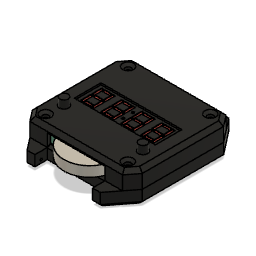
Digital_Watch_Case (Autodesk Fusion 360 design; units mm, degrees)
Autodesk Fusion 360 part; units mm, degrees
sketch "Sketch1" plane through (0, 0, 0) normal (0, 1, 0) x (1, 0, 0)
  line L0 (0, 0) -> (0, 18.5)
  line L1 (0, 18.5) -> (19.75, 18.5)
  line L2 (19.75, 18.5) -> (-19.75, 18.5)
  line L3 (-19.75, 18.5) -> (-19.75, -18.5)
  line L4 (-19.75, -18.5) -> (19.75, -18.5)
  line L5 (19.75, -18.5) -> (19.75, 18.5)
  line L6 (0, 18.5) -> (0, 5.15)
  line L7 (19.75, 0) -> (15.95, 0)
  line L8 (-19.75, 0) -> (-15.95, 0)
  line L9 (0, 5.15) -> (0, -5.05)
  line L10 (-15.95, 0) -> (-15.95, 5.15)
  line L11 (-15.95, 5.15) -> (15.95, 5.15)
  line L12 (15.95, 5.15) -> (15.95, -5.05)
  line L13 (15.95, -5.05) -> (-15.95, -5.05)
  line L14 (-15.95, -5.05) -> (-15.95, 5.15)
  circle A0 centre (0, -15.3) radius 10.25
  line L15 (15.95, -5.05) -> (15.95, -9.75)
  line L16 (19.75, -9.75) -> (15.75, -9.75)
  circle A1 centre (15.75, -9.75) radius 1.665
  circle A2 centre (-15.75, -9.75) radius 1.665
  line L17 (19.75, 18.5) -> (19.75, 17.8)
  line L18 (19.75, 17.8) -> (17.75, 17.8)
  line L19 (17.75, 17.8) -> (15.05, 17.8)
  line L20 (15.05, 17.8) -> (15.05, 15.1)
  line L21 (15.05, 15.1) -> (17.75, 15.1)
  line L22 (17.75, 15.1) -> (17.75, 17.8)
  circle A3 centre (16.4, 16.45) radius 1.35
  circle A4 centre (-16.4, 16.45) radius 1.35
  circle A5 centre (16.4, -16.45) radius 1.35
  circle A6 centre (-16.4, -16.45) radius 1.35
  line L23 (19.75, 18.5) -> (19.75, 15.5)
  line L24 (19.75, 18.5) -> (17.42, 18.5)
  line L25 (17.42, 18.5) -> (19.75, 15.5)
  line L26 (-17.42, 18.5) -> (-19.75, 15.5)
  line L27 (-17.42, -18.5) -> (-19.75, -15.5)
  line L28 (17.42, -18.5) -> (19.75, -15.5)
  line L29 (19.75, 5.15) -> (-19.75, 5.15)
  line L30 (-19.75, 5.15) -> (-19.75, 13.65)
  line L31 (-19.75, 13.65) -> (19.75, 13.65)
  line L32 (19.75, 13.65) -> (19.75, 5.15)
  line L33 (-19.75, 13.65) -> (-9.75, 13.65)
  line L34 (-9.75, 13.65) -> (-19.75, 13.65)
  line L35 (-19.75, 13.65) -> (-19.75, 5.15)
  line L36 (-19.75, 5.15) -> (-9.75, 5.15)
  line L37 (-9.75, 5.15) -> (-9.75, 13.65)
  line L38 (19.75, 13.65) -> (-6.25, 13.65)
  line L39 (-6.25, 13.65) -> (-6.25, 5.15)
  line L40 (-6.25, 5.15) -> (19.75, 5.15)
  line L41 (19.75, 5.15) -> (19.75, 13.65)
  line L42 (19.75, 5.15) -> (19.7, 5.15)
  line L43 (19.7, 5.15) -> (19.7, 5.2)
  line L44 (19.7, 5.2) -> (19.7, 13.65)
  line L45 (-19.75, 5.15) -> (-19.7, 5.15)
  line L46 (-19.7, 5.15) -> (-19.7, 13.65)
  dimension "d1" = 18.5
  dimension "d2" = 19.75
  dimension "d3" = 39.5
  dimension "d4" = 37
  dimension "d5" = 13.35
  dimension "d6" = 3.8
  dimension "d7" = 3.8
  dimension "d8" = 10.2
  dimension "d9" = 20.5
  dimension "d10" = 4.7
  dimension "d11" = 4
  dimension "d12" = 3.33
  dimension "d13" = 0.7
  dimension "d14" = 2
  dimension "d15" = 2.7
  dimension "d16" = 2.7
  dimension "d17" = 3
  dimension "d18" = 2.33
  dimension "d27" = 8.5
  dimension "d28" = 10
  dimension "d29" = 26
  dimension "d32" = 0.05
  dimension "d33" = 180
  dimension "d34" = 0.05
  constraint coincident L0.start origin
  constraint vertical L0
  constraint perpendicular L0 L1
  constraint horizontal L2
  constraint vertical L3
  constraint horizontal L4
  constraint vertical L5
  constraint perpendicular L2 L6
  constraint midpoint L5 L7.start
  constraint perpendicular L5 L7
  constraint midpoint L3 L8.start
  constraint perpendicular L3 L8
  constraint parallel L6 L9
  constraint perpendicular L8 L10
  constraint horizontal L11
  constraint vertical L12
  constraint horizontal L13
  constraint vertical L14
  constraint coincident L9.end A0
  constraint perpendicular L13 L15
  constraint coincident L5 L16.start
  constraint perpendicular L15 L16
  constraint coincident L16.end A1.centre
  constraint symmetric L9 A1 A2
  constraint perpendicular L2 L17
  constraint perpendicular L17 L18
  constraint horizontal L19
  constraint vertical L20
  constraint horizontal L21
  constraint vertical L22
  constraint tangent L22 A3
  constraint symmetric L0 A3 A4
  constraint symmetric L7 A3 A5
  constraint symmetric L7 A4 A6
  constraint perpendicular L18 L23
  constraint perpendicular L23 L24
  constraint symmetric L0 L23.end L26.end
  constraint symmetric L0 L24.end L26.start
  constraint symmetric L7 L23.end L28.end
  constraint symmetric L7 L24.end L28.start
  constraint symmetric L7 L26.start L27.start
  constraint symmetric L7 L26.end L27.end
  constraint horizontal L29
  constraint vertical L30
  constraint horizontal L31
  constraint vertical L32
  constraint coincident L5 L29.start
  constraint perpendicular L30 L33
  constraint horizontal L34
  constraint vertical L35
  constraint horizontal L36
  constraint vertical L37
  constraint horizontal L38
  constraint vertical L39
  constraint horizontal L40
  constraint vertical L41
  constraint horizontal L42
  constraint perpendicular L29 L43
  constraint perpendicular L35 L45
  constraint vertical L46
  measures "d1" distance of L0.start L0.end
  measures "d2" distance of L0.end L1.end
  measures "d3" distance of L1.end L2.end
  measures "d4" distance of L1.end L4.end
  measures "d5" distance of L0.end L6.end
  measures "d6" distance of L7.start L7.end
  measures "d7" distance of L8.start L8.end
  measures "d8" distance of L6.end L9.end
  measures "d9" diameter of A0
  measures "d10" distance of L12.end L15.end
  measures "d11" distance of L16.start L16.end
  measures "d12" diameter of A1
  measures "d13" distance of L1.end L17.end
  measures "d14" distance of L17.end L18.end
  measures "d15" distance of L18.end L19.end
  measures "d16" distance of L18.end L21.end
  measures "d17" distance of L1.end L23.end
  measures "d18" distance of L1.end L24.end
  measures "d27" distance of L29.start L31.end
  measures "d28" distance of L30.end L33.end
  measures "d29" distance of L31.end L38.end
  measures "d32" distance of L29.start L42.end
  measures "d33" angle of L43 L44
  measures "d34" distance of L29.end L45.end
extrude "Extrude1" add sketch "Sketch1" against normal blind 1.7 contours L0 L9 L10 L11 L13 L14 L29 L36 L40 | L0 L9 L11 L12 L13 L29 L40 | L0 L6 L11 L29 L31 L38 L39 L40 | L0 L6 L11 L29 L31 L38 L40 L43 L44 | L3 L4 L8 L13 L14 A0 L27 | L4 L5 L13 A0 L15 L16 A1 L28 | L4 A0 | L0 L2 L3 L6 L26 L31 L33 L34 L38 | L0 L1 L2 L5 L6 L25 L31 L38 | L11 L29 L31 L37 L39 | L5 L7 L12 L29 L40 L42 | L5 L7 L12 L15 L16 A1 | L5 L29 L31 L32 L38 L40 L41 L42 L43 L44 | L11 L29 L31 L33 L34 L36 L37 L46 | L15 L16 A1 | L15 L16 A1 | L3 L8 L10 L14 L29 L36 L45 | L3 L29 L30 L31 L33 L34 L35 L36 L45 L46 | A2 | L19 L22 A3 | L19 L20 A3 | L21 L22 A3 | L20 L21 A3 picked at (3.2783, -16.4707) makes body 1
extrude "Extrude2" add sketch "Sketch1" along normal blind 4 contours L4 A0 | L4 A0 bodies 1
extrude "Extrude3" add sketch "Sketch1" along normal blind 10 contours L15 L16 A1 | L15 L16 A1 | A2 bodies 1
extrude "Extrude4" add sketch "Sketch1" along normal blind 6.5 separate body contours L0 L9 L10 L11 L13 L14 L29 L36 L40 | L0 L9 L11 L12 L13 L29 L40 makes body 2
extrude "Extrude5" add sketch "Sketch1" along normal blind 4 contours L0 L6 L11 L29 L31 L38 L39 L40 | L0 L6 L11 L29 L31 L38 L40 L43 L44 | L11 L29 L31 L33 L34 L36 L37 L46 bodies 1 2
sketch "Sketch10" plane through (0, 6.5, 0) normal (0, 1, 0) x (-1, 0, 0)
  line L0 (15.95, 5.05) -> (-15.95, 5.05)
  line L1 (-15.95, 5.05) -> (-15.95, -5.15)
  line L2 (-15.95, -5.15) -> (15.95, -5.15)
  line L3 (15.95, -5.15) -> (15.95, 5.05)
  line L4 (0, 0) -> (7.975, 0)
  line L5 (7.975, 0) -> (7.975, -5.15)
  line L6 (7.975, 0) -> (7.975, 5.05)
  line L7 (7.975, 0) -> (11.9625, 0)
  line L8 (11.9625, 0) -> (11.9625, -0.5)
  line L9 (11.9625, -0.5) -> (10.4625, -0.5)
  line L10 (10.4625, -0.5) -> (13.4625, -0.5)
  line L11 (13.4625, -0.5) -> (13.4625, 0.5)
  line L12 (13.4625, 0.5) -> (10.4625, 0.5)
  line L13 (10.4625, 0.5) -> (10.4625, -0.5)
  line L14 (10.4625, 0) -> (10.2625, 0)
  line L15 (10.2625, 0) -> (10.2625, -0.2)
  line L16 (10.2625, -0.2) -> (10.4625, -0.2)
  line L17 (10.4625, -0.2) -> (10.4625, 0)
  line L18 (10.4625, 0) -> (10.2625, 0)
  line L19 (10.2625, 0) -> (10.2625, 0.2)
  line L20 (10.2625, 0.2) -> (10.4625, 0.2)
  line L21 (10.4625, 0.2) -> (10.4625, 0)
  line L22 (10.2625, 0.2) -> (9.2625, 0.2)
  line L23 (9.2625, 0.2) -> (9.2625, 4.2)
  line L24 (9.2625, 4.2) -> (10.2625, 4.2)
  line L25 (10.2625, 4.2) -> (10.2625, 0.2)
  line L26 (10.2625, -0.2) -> (9.2625, -0.2)
  line L27 (9.2625, -0.2) -> (9.2625, -4.2)
  line L28 (9.2625, -4.2) -> (10.2625, -4.2)
  line L29 (10.2625, -4.2) -> (10.2625, -0.2)
  line L30 (10.2625, 4.2) -> (10.4625, 4.2)
  line L31 (10.4625, 4.2) -> (13.4625, 4.2)
  line L32 (13.4625, 4.2) -> (13.4625, 3.2)
  line L33 (13.4625, 3.2) -> (10.4625, 3.2)
  line L34 (10.4625, 3.2) -> (10.4625, 4.2)
  line L35 (13.4625, 0) -> (13.6625, 0)
  line L36 (13.6625, 0) -> (13.6625, 0.2)
  line L37 (13.6625, 0.2) -> (13.4625, 0.2)
  line L38 (13.4625, 0.2) -> (13.4625, 0)
  line L39 (13.4625, 0) -> (13.6625, 0)
  line L40 (13.6625, 0) -> (13.6625, -0.2)
  line L41 (13.6625, -0.2) -> (13.4625, -0.2)
  line L42 (13.4625, -0.2) -> (13.4625, 0)
  line L43 (13.6625, -0.2) -> (14.6625, -0.2)
  line L44 (14.6625, -0.2) -> (14.6625, -4.2)
  line L45 (14.6625, -4.2) -> (13.6625, -4.2)
  line L46 (13.6625, -4.2) -> (13.6625, -0.2)
  line L47 (13.6625, 0.2) -> (14.6625, 0.2)
  line L48 (14.6625, 0.2) -> (14.6625, 4.2)
  line L49 (14.6625, 4.2) -> (13.6625, 4.2)
  line L50 (13.6625, 4.2) -> (13.6625, 0.2)
  line L51 (13.6625, -4.2) -> (13.4625, -4.2)
  line L52 (13.4625, -4.2) -> (10.4625, -4.2)
  line L53 (10.4625, -4.2) -> (10.4625, -3.2)
  line L54 (10.4625, -3.2) -> (13.4625, -3.2)
  line L55 (13.4625, -3.2) -> (13.4625, -4.2)
  line L56 (1.2875, 0.2) -> (1.2875, 4.2)
  line L57 (6.6875, 0.2) -> (6.6875, 4.2)
  line L58 (5.6875, 0.2) -> (5.4875, 0.2)
  line L59 (2.2875, -4.2) -> (2.4875, -4.2)
  line L60 (2.4875, -0.2) -> (2.4875, 0)
  line L61 (2.4875, -0.5) -> (2.4875, 0.5)
  line L62 (2.2875, -4.2) -> (2.2875, -0.2)
  line L63 (5.4875, 0) -> (5.6875, 0)
  line L64 (2.2875, 0) -> (2.2875, 0.2)
  line L65 (2.4875, 0) -> (2.2875, 0)
  line L66 (2.2875, -0.2) -> (2.4875, -0.2)
  line L67 (2.2875, 0.2) -> (1.2875, 0.2)
  line L68 (5.6875, 0) -> (5.6875, 0.2)
  line L69 (5.4875, -0.5) -> (2.4875, -0.5)
  line L70 (2.4875, 0) -> (2.2875, 0)
  line L71 (2.4875, 0.2) -> (2.4875, 0)
  line L72 (5.4875, -3.2) -> (2.4875, -3.2)
  line L73 (5.4875, 0) -> (5.6875, 0)
  line L74 (5.4875, -0.2) -> (5.4875, 0)
  line L75 (5.4875, 4.2) -> (2.4875, 4.2)
  line L76 (6.6875, -0.2) -> (6.6875, -4.2)
  line L77 (1.2875, 4.2) -> (2.2875, 4.2)
  line L78 (6.6875, -4.2) -> (5.6875, -4.2)
  line L79 (5.6875, 4.2) -> (5.6875, 0.2)
  line L80 (2.2875, 4.2) -> (2.2875, 0.2)
  line L81 (2.4875, 4.2) -> (2.4875, 3.2)
  line L82 (5.6875, -0.2) -> (6.6875, -0.2)
  line L83 (5.4875, 3.2) -> (5.4875, 4.2)
  line L84 (5.4875, -4.2) -> (5.4875, -3.2)
  line L85 (6.6875, 4.2) -> (5.6875, 4.2)
  line L86 (2.4875, 3.2) -> (5.4875, 3.2)
  line L87 (5.6875, 4.2) -> (5.4875, 4.2)
  line L88 (5.6875, 0.2) -> (6.6875, 0.2)
  line L89 (2.2875, -0.2) -> (1.2875, -0.2)
  line L90 (2.2875, 0) -> (2.2875, -0.2)
  line L91 (5.6875, -0.2) -> (5.4875, -0.2)
  line L92 (5.4875, 0.5) -> (5.4875, -0.5)
  line L93 (5.4875, 0.2) -> (5.4875, 0)
  line L94 (2.4875, -3.2) -> (2.4875, -4.2)
  line L95 (2.2875, 0.2) -> (2.4875, 0.2)
  line L96 (5.6875, 0) -> (5.6875, -0.2)
  line L97 (2.4875, -4.2) -> (5.4875, -4.2)
  line L98 (3.9875, 0) -> (3.9875, -0.5)
  line L99 (1.2875, -4.2) -> (2.2875, -4.2)
  line L100 (1.2875, -0.2) -> (1.2875, -4.2)
  line L101 (2.4875, 0.5) -> (5.4875, 0.5)
  line L102 (3.9875, -0.5) -> (5.4875, -0.5)
  line L103 (5.6875, -4.2) -> (5.6875, -0.2)
  line L104 (0, 0) -> (0, -5.15)
  line L105 (-9.2625, 0.2) -> (-9.2625, 4.2)
  line L106 (-1.2875, 0.2) -> (-1.2875, 4.2)
  line L107 (-14.6625, 0.2) -> (-14.6625, 4.2)
  line L108 (-10.2625, 4.2) -> (-10.2625, 0.2)
  line L109 (-5.4875, -3.2) -> (-2.4875, -3.2)
  line L110 (-10.4625, -0.5) -> (-13.4625, -0.5)
  line L111 (-3.9875, 0) -> (-3.9875, -0.5)
  line L112 (-13.4625, 3.2) -> (-10.4625, 3.2)
  line L113 (-5.4875, -0.5) -> (-2.4875, -0.5)
  line L114 (-10.4625, 0) -> (-10.2625, 0)
  line L115 (-5.4875, 0) -> (-5.6875, 0)
  line L116 (-2.2875, -4.2) -> (-2.4875, -4.2)
  line L117 (-10.4625, 3.2) -> (-10.4625, 4.2)
  line L118 (-11.9625, 0) -> (-11.9625, -0.5)
  line L119 (-1.2875, 4.2) -> (-2.2875, 4.2)
  line L120 (-2.4875, 0.2) -> (-2.4875, 0)
  line L121 (-3.9875, -0.5) -> (-5.4875, -0.5)
  line L122 (-10.4625, 4.2) -> (-13.4625, 4.2)
  line L123 (-7.975, 0) -> (-11.9625, 0)
  line L124 (-5.4875, 4.2) -> (-2.4875, 4.2)
  line L125 (-10.2625, 4.2) -> (-10.4625, 4.2)
  line L126 (-5.6875, 4.2) -> (-5.4875, 4.2)
  line L127 (-5.6875, 4.2) -> (-5.6875, 0.2)
  line L128 (-13.6625, 4.2) -> (-13.6625, 0.2)
  line L129 (-6.6875, 0.2) -> (-6.6875, 4.2)
  line L130 (-10.2625, -0.2) -> (-9.2625, -0.2)
  line L131 (-2.2875, 4.2) -> (-2.2875, 0.2)
  line L132 (-2.4875, 4.2) -> (-2.4875, 3.2)
  line L133 (-5.4875, 0.2) -> (-5.4875, 0)
  line L134 (-10.2625, 0) -> (-10.2625, 0.2)
  line L135 (-11.9625, -0.5) -> (-10.4625, -0.5)
  line L136 (-10.4625, 0.2) -> (-10.4625, 0)
  line L137 (-13.4625, 4.2) -> (-13.4625, 3.2)
  line L138 (-2.4875, 0.5) -> (-5.4875, 0.5)
  line L139 (-5.4875, -0.2) -> (-5.4875, 0)
  line L140 (-6.6875, 4.2) -> (-5.6875, 4.2)
  line L141 (-13.6625, 0) -> (-13.6625, 0.2)
  line L142 (-2.4875, -4.2) -> (-5.4875, -4.2)
  line L143 (-13.6625, -4.2) -> (-13.6625, -0.2)
  line L144 (-10.4625, -3.2) -> (-13.4625, -3.2)
  line L145 (-5.6875, 0.2) -> (-5.4875, 0.2)
  line L146 (-9.2625, 4.2) -> (-10.2625, 4.2)
  line L147 (-1.2875, -0.2) -> (-1.2875, -4.2)
  line L148 (-13.4625, -3.2) -> (-13.4625, -4.2)
  line L149 (-2.4875, 3.2) -> (-5.4875, 3.2)
  line L150 (-2.2875, 0) -> (-2.2875, 0.2)
  line L151 (-13.4625, 0) -> (-13.6625, 0)
  line L152 (-5.4875, 3.2) -> (-5.4875, 4.2)
  line L153 (-14.6625, 4.2) -> (-13.6625, 4.2)
  line L154 (-5.6875, -0.2) -> (-5.4875, -0.2)
  line L155 (-9.2625, -4.2) -> (-10.2625, -4.2)
  line L156 (-10.2625, 0.2) -> (-9.2625, 0.2)
  line L157 (-10.2625, -4.2) -> (-10.2625, -0.2)
  line L158 (-2.2875, -4.2) -> (-2.2875, -0.2)
  line L159 (-9.2625, -0.2) -> (-9.2625, -4.2)
  line L160 (-10.4625, -0.2) -> (-10.4625, 0)
  line L161 (-6.6875, -4.2) -> (-5.6875, -4.2)
  line L162 (-13.6625, -0.2) -> (-13.4625, -0.2)
  line L163 (-10.2625, 0) -> (-10.2625, -0.2)
  line L164 (-10.2625, 0.2) -> (-10.4625, 0.2)
  line L165 (-13.4625, -0.5) -> (-13.4625, 0.5)
  line L166 (-2.2875, 0) -> (-2.2875, -0.2)
  line L167 (-10.2625, -0.2) -> (-10.4625, -0.2)
  line L168 (-13.6625, 0.2) -> (-13.4625, 0.2)
  line L169 (-13.6625, 0) -> (-13.6625, -0.2)
  line L170 (-13.4625, 0.2) -> (-13.4625, 0)
  line L171 (-14.6625, -4.2) -> (-13.6625, -4.2)
  line L172 (-14.6625, -0.2) -> (-14.6625, -4.2)
  line L173 (-5.6875, 0.2) -> (-6.6875, 0.2)
  line L174 (-5.6875, 0) -> (-5.6875, 0.2)
  line L175 (-13.6625, 0.2) -> (-14.6625, 0.2)
  line L176 (-10.4625, 0) -> (-10.2625, 0)
  line L177 (-13.6625, -0.2) -> (-14.6625, -0.2)
  line L178 (-5.4875, 0) -> (-5.6875, 0)
  line L179 (-2.4875, 0) -> (-2.2875, 0)
  line L180 (-5.4875, -4.2) -> (-5.4875, -3.2)
  line L181 (-2.4875, 0) -> (-2.2875, 0)
  line L182 (-2.2875, 0.2) -> (-2.4875, 0.2)
  line L183 (-5.6875, -4.2) -> (-5.6875, -0.2)
  line L184 (-10.4625, -4.2) -> (-10.4625, -3.2)
  line L185 (-5.6875, -0.2) -> (-6.6875, -0.2)
  line L186 (-5.6875, 0) -> (-5.6875, -0.2)
  line L187 (-5.4875, 0.5) -> (-5.4875, -0.5)
  line L188 (-2.4875, -0.5) -> (-2.4875, 0.5)
  line L189 (-2.2875, -0.2) -> (-1.2875, -0.2)
  line L190 (-13.4625, -4.2) -> (-10.4625, -4.2)
  line L191 (-2.4875, -0.2) -> (-2.4875, 0)
  line L192 (-13.6625, -4.2) -> (-13.4625, -4.2)
  line L193 (-10.4625, 0.5) -> (-10.4625, -0.5)
  line L194 (-6.6875, -0.2) -> (-6.6875, -4.2)
  line L195 (-2.2875, -0.2) -> (-2.4875, -0.2)
  line L196 (-2.2875, 0.2) -> (-1.2875, 0.2)
  line L197 (-13.4625, 0) -> (-13.6625, 0)
  line L198 (-2.4875, -3.2) -> (-2.4875, -4.2)
  line L199 (-13.4625, 0.5) -> (-10.4625, 0.5)
  line L200 (-13.4625, -0.2) -> (-13.4625, 0)
  line L201 (-1.2875, -4.2) -> (-2.2875, -4.2)
  line L202 (0, 0) -> (0, -2)
  circle A0 centre (0, -2) radius 0.5
  line L203 (0, 0) -> (0, 2)
  circle A1 centre (0, 2) radius 0.5
  dimension "d101" = 7.975
  dimension "d102" = 3.9875
  dimension "d103" = 1.5
  dimension "d104" = 3
  dimension "d105" = 0.2
  dimension "d106" = 0.2
  dimension "d107" = 0.2
  dimension "d108" = 1
  dimension "d109" = 4
  dimension "d110" = 1
  dimension "d111" = 4
  dimension "d112" = 0.2
  dimension "d113" = 3
  dimension "d114" = 1
  dimension "d115" = 0.2
  dimension "d116" = 0.2
  dimension "d117" = 0.2
  dimension "d118" = 0.2
  dimension "d119" = 1
  dimension "d120" = 4
  dimension "d121" = 1
  dimension "d122" = 4
  dimension "d123" = 0.2
  dimension "d124" = 3
  dimension "d125" = 1
  dimension "d126" = 1
  dimension "d127" = 2
  dimension "d128" = 1
  constraint coincident L4.start L104.start
  constraint perpendicular L3 L4
  constraint coincident L2 L5.end
  constraint perpendicular L2 L5
  constraint coincident L0 L6.end
  constraint perpendicular L0 L6
  constraint perpendicular L3 L7
  constraint perpendicular L7 L8
  constraint perpendicular L8 L9
  constraint horizontal L10
  constraint vertical L11
  constraint horizontal L12
  constraint vertical L13
  constraint horizontal L14
  constraint vertical L15
  constraint horizontal L16
  constraint vertical L17
  constraint midpoint L13 L14.start
  constraint horizontal L18
  constraint vertical L19
  constraint horizontal L20
  constraint vertical L21
  constraint horizontal L22
  constraint vertical L23
  constraint horizontal L24
  constraint vertical L25
  constraint horizontal L26
  constraint vertical L27
  constraint horizontal L28
  constraint vertical L29
  constraint perpendicular L25 L30
  constraint horizontal L31
  constraint vertical L32
  constraint horizontal L33
  constraint vertical L34
  constraint horizontal L35
  constraint vertical L36
  constraint horizontal L37
  constraint vertical L38
  constraint midpoint L11 L35.start
  constraint horizontal L39
  constraint vertical L40
  constraint horizontal L41
  constraint vertical L42
  constraint horizontal L43
  constraint vertical L44
  constraint horizontal L45
  constraint vertical L46
  constraint horizontal L47
  constraint vertical L48
  constraint horizontal L49
  constraint vertical L50
  constraint perpendicular L46 L51
  constraint horizontal L52
  constraint vertical L53
  constraint horizontal L54
  constraint vertical L55
  constraint symmetric L5 L7.end L98.start
  constraint symmetric L5 L8.end L98.end
  constraint symmetric L5 L9.end L69.start
  constraint symmetric L5 L10.end L61.start
  constraint symmetric L5 L11.end L61.end
  constraint symmetric L5 L12.end L92.start
  constraint symmetric L5 L14.start L63.start
  constraint symmetric L5 L14.end L63.end
  constraint symmetric L5 L15.end L82.start
  constraint symmetric L5 L16.end L74.start
  constraint symmetric L5 L19.end L58.start
  constraint symmetric L5 L20.end L58.end
  constraint symmetric L5 L22.end L57.start
  constraint symmetric L5 L23.end L57.end
  constraint symmetric L5 L24.end L79.start
  constraint symmetric L5 L26.end L76.start
  constraint symmetric L5 L27.end L76.end
  constraint symmetric L5 L28.end L78.end
  constraint symmetric L5 L30.end L75.start
  constraint symmetric L5 L31.end L75.end
  constraint symmetric L5 L32.end L81.end
  constraint symmetric L5 L33.end L83.start
  constraint symmetric L5 L35.start L60.end
  constraint symmetric L5 L35.end L64.start
  constraint symmetric L5 L36.end L64.end
  constraint symmetric L5 L37.end L71.start
  constraint symmetric L5 L40.end L62.end
  constraint symmetric L5 L41.end L60.start
  constraint symmetric L5 L43.end L89.end
  constraint symmetric L5 L44.end L99.start
  constraint symmetric L5 L45.end L59.start
  constraint symmetric L5 L47.end L56.start
  constraint symmetric L5 L48.end L56.end
  constraint symmetric L5 L49.end L77.end
  constraint symmetric L5 L51.end L59.end
  constraint symmetric L5 L52.end L84.start
  constraint symmetric L5 L53.end L72.start
  constraint symmetric L5 L54.end L72.end
  constraint midpoint L2 L104.end
  constraint symmetric L4.end L104 L123.start
  constraint symmetric L7.end L104 L118.start
  constraint symmetric L8.end L104 L118.end
  constraint symmetric L9.end L104 L110.start
  constraint symmetric L10.end L104 L110.end
  constraint symmetric L11.end L104 L165.end
  constraint symmetric L12.end L104 L193.start
  constraint symmetric L14.start L104 L114.start
  constraint symmetric L14.end L104 L114.end
  constraint symmetric L15.end L104 L130.start
  constraint symmetric L16.end L104 L160.start
  constraint symmetric L19.end L104 L108.end
  constraint symmetric L20.end L104 L136.start
  constraint symmetric L22.end L104 L105.start
  constraint symmetric L23.end L104 L105.end
  constraint symmetric L24.end L104 L108.start
  constraint symmetric L26.end L104 L130.end
  constraint symmetric L27.end L104 L155.start
  constraint symmetric L28.end L104 L155.end
  constraint symmetric L30.end L104 L117.end
  constraint symmetric L31.end L104 L122.end
  constraint symmetric L32.end L104 L112.start
  constraint symmetric L33.end L104 L112.end
  constraint symmetric L35.start L104 L151.start
  constraint symmetric L35.end L104 L141.start
  constraint symmetric L36.end L104 L128.end
  constraint symmetric L37.end L104 L168.end
  constraint symmetric L40.end L104 L143.end
  constraint symmetric L41.end L104 L162.end
  constraint symmetric L43.end L104 L172.start
  constraint symmetric L44.end L104 L171.start
  constraint symmetric L45.end L104 L143.start
  constraint symmetric L47.end L104 L107.start
  constraint symmetric L48.end L104 L107.end
  constraint symmetric L49.end L104 L128.start
  constraint symmetric L51.end L104 L148.end
  constraint symmetric L52.end L104 L184.start
  constraint symmetric L53.end L104 L144.start
  constraint symmetric L54.end L104 L144.end
  constraint symmetric L84.start L104 L142.end
  constraint symmetric L99.start L104 L147.end
  constraint symmetric L59.start L104 L116.start
  constraint symmetric L78.end L104 L161.end
  constraint symmetric L72.end L104 L109.end
  constraint symmetric L72.start L104 L109.start
  constraint symmetric L76.end L104 L161.start
  constraint symmetric L59.end L104 L116.end
  constraint symmetric L64.start L104 L150.start
  constraint symmetric L71.start L104 L120.start
  constraint symmetric L62.end L104 L158.end
  constraint symmetric L83.start L104 L149.end
  constraint symmetric L56.end L104 L106.end
  constraint symmetric L56.start L104 L106.start
  constraint symmetric L64.end L104 L131.end
  constraint symmetric L60.end L104 L120.end
  constraint symmetric L89.end L104 L147.start
  constraint symmetric L60.start L104 L191.start
  constraint symmetric L69.start L104 L113.start
  constraint symmetric L98.end L104 L111.end
  constraint symmetric L98.start L104 L111.start
  constraint symmetric L61.end L104 L138.start
  constraint symmetric L61.start L104 L113.end
  constraint symmetric L92.start L104 L138.end
  constraint symmetric L58.start L104 L127.end
  constraint symmetric L63.start L104 L115.start
  constraint symmetric L74.start L104 L139.start
  constraint symmetric L82.start L104 L154.start
  constraint symmetric L63.end L104 L115.end
  constraint symmetric L58.end L104 L133.start
  constraint symmetric L79.start L104 L126.start
  constraint symmetric L75.start L104 L124.start
  constraint symmetric L81.end L104 L132.end
  constraint symmetric L77.end L104 L119.end
  constraint symmetric L76.start L104 L185.end
  constraint symmetric L75.end L104 L124.end
  constraint symmetric L57.end L104 L129.end
  constraint symmetric L57.start L104 L129.start
  constraint coincident L104 L202.end
  constraint coincident L202.end A0.centre
  constraint perpendicular L4 L203
  constraint coincident L203.end A1.centre
  measures "d101" distance of L4.start L4.end
  measures "d102" distance of L4.end L7.end
  measures "d103" distance of L8.end L9.end
  measures "d104" distance of L9.end L10.end
  measures "d105" distance of L14.start L14.end
  measures "d106" distance of L14.start L16.end
  measures "d107" distance of L14.start L20.end
  measures "d108" distance of L19.end L22.end
  measures "d109" distance of L19.end L24.end
  measures "d110" distance of L15.end L26.end
  measures "d111" distance of L15.end L28.end
  measures "d112" distance of L24.end L30.end
  measures "d113" distance of L30.end L31.end
  measures "d114" distance of L30.end L33.end
  measures "d115" distance of L35.start L35.end
  measures "d116" distance of L35.start L37.end
  measures "d117" distance of L35.start L35.end
  measures "d118" distance of L35.start L41.end
  measures "d119" distance of L40.end L43.end
  measures "d120" distance of L40.end L45.end
  measures "d121" distance of L36.end L47.end
  measures "d122" distance of L36.end L49.end
  measures "d123" distance of L45.end L51.end
  measures "d124" distance of L51.end L52.end
  measures "d125" distance of L51.end L54.end
  measures "d126" diameter of A0
  measures "d127" distance of L4.start L203.end
  measures "d128" diameter of A1
extrude "Extrude17" cut sketch "Sketch10" against normal blind 0.2 contours L56 L67 L77 L80 | L57 L79 L85 L88 | L76 L78 L82 L103 | L62 L89 L99 L100 | L4 L69 L74 L92 L98 L102 | L4 L61 L71 L92 L93 L101 | L104 L202 A0 | L104 L202 A0 | L4 L60 L61 L69 L98 | L22 L23 L24 L25 | L47 L48 L49 L50 | L43 L44 L45 L46 | L26 L27 L28 L29 | L7 L8 L10 L11 L12 L13 L21 L38 L42 | L7 L8 L9 L10 L13 L17 | L31 L32 L33 L34 | L52 L53 L54 L55 | L72 L84 L94 L97 | L75 L81 L83 L86 | L105 L108 L146 L156 | L130 L155 L157 L159 | L143 L171 L172 L177 | L107 L128 L153 L175 | L110 L118 L123 L136 L165 L170 L193 L199 L200 | L110 L118 L123 L135 L160 L193 | L106 L119 L131 L196 | L147 L158 L189 L201 | L161 L183 L185 L194 | L127 L129 L140 L173 | L113 L120 L121 L133 L138 L139 L187 L188 L191 | L109 L142 L180 L198 | L112 L117 L122 L137 | L124 L132 L149 L152 | L144 L148 L184 L190 | A1 bodies 1
sketch "Sketch2" plane through (0, -1.7, 0) normal (0, -1, 0) x (1, 0, 0)
  circle A0 centre (16.4, -16.45) radius 1.35
  circle A1 centre (16.4, 16.45) radius 1.35
  circle A2 centre (-16.4, 16.45) radius 1.35
  circle A3 centre (-16.4, -16.45) radius 1.35
  line L0 (17.42, 18.5) -> (-17.42, 18.5)
  line L1 (-17.42, 18.5) -> (-19.75, 15.5)
  line L2 (-19.75, 15.5) -> (-19.75, -15.5)
  line L3 (-19.75, -15.5) -> (-17.42, -18.5)
  line L4 (-17.42, -18.5) -> (17.42, -18.5)
  line L5 (17.42, -18.5) -> (19.75, -15.5)
  line L6 (19.75, -15.5) -> (19.75, 15.5)
  line L7 (19.75, 15.5) -> (17.42, 18.5)
  line L8 (19.75, -15.5) -> (19.9, -15.5)
  line L9 (17.42, -18.5) -> (17.42, -18.65)
  line L10 (17.42, -18.65) -> (20.7, -18.65)
  line L11 (19.9, -15.5) -> (19.9, -18.9)
  line L12 (-17.42, 18.5) -> (-17.42, 18.65)
  line L13 (-19.75, 15.5) -> (-19.9, 15.5)
  line L14 (-19.9, 15.5) -> (-19.9, 19.2)
  line L15 (-17.42, 18.65) -> (-20.3, 18.65)
  line L16 (-19.9, 18.65) -> (19.9, 18.65)
  line L17 (19.9, 18.65) -> (19.9, -18.65)
  line L18 (19.9, -18.65) -> (-19.9, -18.65)
  line L19 (-19.9, -18.65) -> (-19.9, 18.65)
  circle A4 centre (16.4, 16.45) radius 2
  circle A5 centre (16.4, -16.45) radius 2
  circle A6 centre (-16.4, -16.45) radius 2
  circle A7 centre (-16.4, 16.45) radius 2
  line L20 (-21.9, -20.65) -> (-21.9, 20.65)
  line L21 (-21.9, 20.65) -> (21.9, 20.65)
  line L22 (21.9, 20.65) -> (21.9, -20.65)
  line L23 (21.9, -20.65) -> (-21.9, -20.65)
  line L24 (19.9, 15.5514) -> (17.4934, 18.65)
  line L25 (17.4934, 18.65) -> (-17.4934, 18.65)
  line L26 (-17.4934, 18.65) -> (-19.9, 15.5514)
  line L27 (-19.9, 15.5514) -> (-19.9, -15.5514)
  line L28 (-19.9, -15.5514) -> (-17.4934, -18.65)
  line L29 (-17.4934, -18.65) -> (17.4934, -18.65)
  line L30 (17.4934, -18.65) -> (19.9, -15.5514)
  line L31 (19.9, -15.5514) -> (19.9, 15.5514)
  line L32 (21.9, 16.2368) -> (18.4725, 20.65)
  line L33 (18.4725, 20.65) -> (-18.4725, 20.65)
  line L34 (-18.4725, 20.65) -> (-21.9, 16.2368)
  line L35 (-21.9, 16.2368) -> (-21.9, -16.2368)
  line L36 (-21.9, -16.2368) -> (-18.4725, -20.65)
  line L37 (-18.4725, -20.65) -> (18.4725, -20.65)
  line L38 (18.4725, -20.65) -> (21.9, -16.2368)
  line L39 (21.9, -16.2368) -> (21.9, 16.2368)
  circle A8 centre (16.4, 16.45) radius 1
  circle A9 centre (-16.4, 16.45) radius 1
  circle A10 centre (-16.4, -16.45) radius 1
  circle A11 centre (16.4, -16.45) radius 1
  circle A12 centre (-16.4, 16.45) radius 1.2
  circle A13 centre (-16.4, -16.45) radius 1.2
  circle A14 centre (16.4, -16.45) radius 1.2
  circle A15 centre (16.4, 16.45) radius 1.2
  dimension "d35" = 0.15
  dimension "d38" = 0.15
  dimension "d39" = 0.15
  dimension "d40" = 0.15
  dimension "d41" = 4
  dimension "d42" = 4
  dimension "d43" = 4
  dimension "d44" = 4
  dimension "d45" = -2
  dimension "d46" = 0.15
  dimension "d47" = 2.15
  dimension "d50" = 2
  dimension "d51" = 2
  dimension "d52" = 2
  dimension "d53" = 2
  dimension "d90" = 2.4
  dimension "d91" = 2.4
  dimension "d92" = 2.4
  dimension "d93" = 2.4
  constraint coincident L5.end L6.start
  constraint horizontal L8
  constraint coincident L4.end L5.start
  constraint vertical L9
  constraint perpendicular L9 L10
  constraint perpendicular L10 L11
  constraint coincident L0.end L1.start
  constraint perpendicular L0 L12
  constraint coincident L1.end L2.start
  constraint perpendicular L2 L13
  constraint perpendicular L13 L14
  constraint perpendicular L14 L15
  constraint horizontal L16
  constraint vertical L17
  constraint horizontal L18
  constraint vertical L19
  constraint coincident L10 L17.end
  constraint coincident L11 L17.end
  constraint coincident L14 L16.start
  constraint coincident L15 L16.start
  constraint concentric A1 A4
  constraint concentric A0 A5
  constraint concentric A3 A6
  constraint concentric A2 A7
  constraint concentric A4 A8
  constraint concentric A7 A9
  constraint concentric A6 A10
  constraint concentric A5 A11
  constraint concentric A7 A12
  constraint concentric A10 A13
  constraint concentric A11 A14
  constraint concentric A4 A15
  measures "d35" distance of L5.end L8.end
  measures "d38" distance of L4.end L9.end
  measures "d39" distance of L0.end L12.end
  measures "d40" distance of L1.end L13.end
  measures "d41" diameter of A4
  measures "d42" diameter of A5
  measures "d43" diameter of A6
  measures "d44" diameter of A7
  measures "d50" diameter of A8
  measures "d51" diameter of A9
  measures "d52" diameter of A10
  measures "d53" diameter of A11
  measures "d90" diameter of A12
  measures "d91" diameter of A13
  measures "d92" diameter of A14
  measures "d93" diameter of A15
extrude "Extrude6" add sketch "Sketch2" against normal blind 1.5 separate body contours L10 L11 L14 L15 L16 L17 L21 L22 L25 L31 L32 L33 L34 L38 L39 | L10 L11 L14 L15 L18 L19 L20 L23 L27 L29 L34 L35 L36 L37 L38 | L14 L15 L16 L19 L26 | L16 L17 L24 | L18 L19 L28 | L14 L15 L34 | L10 L11 L17 L18 L30 | L10 L11 L38 makes body 3
extrude "Extrude7" add sketch "Sketch2" along normal blind 2 separate body contours A0 | A1 | A2 | A3 | L10 L11 L14 L15 L16 L17 L21 L22 L25 L31 L32 L33 L34 L38 L39 | L10 L11 L14 L15 L18 L19 L20 L23 L27 L29 L34 L35 L36 L37 L38 | L14 L15 L16 L19 L26 | L16 L17 L24 | L18 L19 L28 | L14 L15 L34 | L10 L11 L17 L18 L30 | L10 L11 L38 | A4 | A5 | A6 | A7 | A12 | A13 | A14 | A15 makes body 4 at (18.3901, -3.0333, -16.6491) makes body 5 at (18.3901, -3.0333, 16.2509) makes body 6 at (-14.4099, -3.0333, -16.6491) makes body 7 at (5.8311, -1.7, -19.9833) makes body 8 at (-14.4099, -3.0333, 16.2509)
sketch "Sketch3" plane through (0, -3.7, 0) normal (0, -1, 0) x (1, 0, 0)
  line L0 (19.9, 15.5514) -> (19.9, -15.5514)
  line L1 (19.9, -15.5514) -> (17.4934, -18.65)
  line L2 (17.4934, -18.65) -> (-17.4934, -18.65)
  line L3 (-17.4934, -18.65) -> (-19.9, -15.5514)
  line L4 (-19.9, -15.5514) -> (-19.9, 15.5514)
  line L5 (-19.9, 15.5514) -> (-17.4934, 18.65)
  line L6 (-17.4934, 18.65) -> (17.4934, 18.65)
  line L7 (17.4934, 18.65) -> (19.9, 15.5514)
  line L8 (21.9, -16.2368) -> (21.9, 16.2368)
  line L9 (21.9, 16.2368) -> (18.4725, 20.65)
  line L10 (18.4725, 20.65) -> (-18.4725, 20.65)
  line L11 (-18.4725, 20.65) -> (-21.9, 16.2368)
  line L12 (-21.9, 16.2368) -> (-21.9, -16.2368)
  line L13 (-21.9, -16.2368) -> (-18.4725, -20.65)
  line L14 (-18.4725, -20.65) -> (18.4725, -20.65)
  line L15 (18.4725, -20.65) -> (21.9, -16.2368)
extrude "Extrude8" add sketch "Sketch3" along normal blind 2 contours L0 L1 L2 L3 L4 L5 L6 L7 | L8 L9 L10 L11 L12 L13 L14 L15 bodies 4 5 6 7 8
combine "Combine1" operation add target body 3 tool bodies 4
sketch "Sketch4" plane through (0, -5.7, 0) normal (0, -1, 0) x (1, 0, 0)
  line L0 (18.4725, -20.65) -> (21.9, -16.2368)
  line L1 (21.9, -16.2368) -> (21.9, 16.2368)
  line L2 (21.9, 16.2368) -> (18.4725, 20.65)
  line L3 (18.4725, 20.65) -> (-18.4725, 20.65)
  line L4 (-18.4725, 20.65) -> (-21.9, 16.2368)
  line L5 (-21.9, 16.2368) -> (-21.9, -16.2368)
  line L6 (-21.9, -16.2368) -> (-18.4725, -20.65)
  line L7 (-18.4725, -20.65) -> (18.4725, -20.65)
  line L8 (-21.9, 0) -> (21.9, 0)
  line L9 (0, 20.65) -> (0, -20.65)
  line L10 (0, 20.65) -> (11, 20.65)
  line L11 (0, 20.65) -> (11.5, 20.65)
  line L12 (11.5, 20.65) -> (11.5, 25.65)
  line L13 (18.4725, 20.65) -> (13.3352, 27.2645)
  line L14 (11.5, 25.65) -> (18, 25.65)
  dimension "d58" = 11
  dimension "d59" = 11.5
  dimension "d60" = 5
  constraint midpoint L5 L8.start
  constraint midpoint L1 L8.end
  constraint midpoint L3 L9.start
  constraint midpoint L7 L9.end
  constraint perpendicular L9 L10
  constraint perpendicular L9 L11
  constraint perpendicular L11 L12
  constraint coincident L2.end L3.start
  constraint parallel L2 L13
  constraint perpendicular L12 L14
  measures "d58" distance of L9.start L10.end
  measures "d59" distance of L9.start L11.end
  measures "d60" distance of L11.end L12.end
extrude "Extrude9" add sketch "Sketch4" against normal blind 5.5 contours L3 L12 L13 L14 bodies 3
sketch "Sketch5" plane through (11.5, 0, 0) normal (-1, 0, 0) x (0, 0, 1)
  line L0 (20.65, -5.7) -> (25.65, -5.7)
  line L1 (25.65, -5.7) -> (25.65, -0.2)
  line L2 (25.65, -0.2) -> (20.65, -0.2)
  line L3 (20.65, -0.2) -> (20.65, -5.7)
  circle A0 centre (23.15, -2.95) radius 0.45
  dimension "d63" = 0.9
  measures "d63" diameter of A0
extrude "Extrude10" cut sketch "Sketch5" against normal blind 1.2 contours A0 bodies 3
mirror "Mirror1" about plane through (0, 0, 0) normal (1, 0, 0) of "Extrude9", "Extrude10"
mirror "Mirror2" about plane through (0, 0, 0) normal (0, 0, 1) of "Extrude9", "Extrude10", "Mirror1"
chamfer "Chamfer1" distance 0.5 angle 45 4 edges at (15.4677, -1.7, -16.0884) (-17.3323, -1.7, -16.0884) (-17.3323, -1.7, 16.8116) (15.4677, -1.7, 16.8116) on bodies 3
chamfer "Chamfer2" distance 1.5 angle 45 16 edges at (-18.2446, -5.7, 20.9434) (-13.0446, -5.7, 25.65) (-11.5, -5.7, 23.15) (0, -5.7, 20.65) (11.5, -5.7, 23.15) (13.0446, -5.7, 25.65) (18.2446, -5.7, 20.9434) (18.2446, -5.7, -20.9434) (13.0446, -5.7, -25.65) (11.5, -5.7, -23.15) (0, -5.7, -20.65) (-11.5, -5.7, -23.15) (-13.0446, -5.7, -25.65) (-18.2446, -5.7, -20.9434) (-21.9, -5.7, 0) (21.9, -5.7, 0) on bodies 3
sketch "Sketch6" plane through (0, -0.2, 0) normal (0, 1, 0) x (-1, 0, 0)
  line L0 (-19.9, -15.5514) -> (-19.9, 15.5514)
  line L1 (-19.9, 15.5514) -> (-17.4934, 18.65)
  line L2 (-17.4934, 18.65) -> (17.4934, 18.65)
  line L3 (17.4934, 18.65) -> (19.9, 15.5514)
  line L4 (19.9, 15.5514) -> (19.9, -15.5514)
  line L5 (19.9, -15.5514) -> (17.4934, -18.65)
  line L6 (17.4934, -18.65) -> (-17.4934, -18.65)
  line L7 (-17.4934, -18.65) -> (-19.9, -15.5514)
  line L8 (-21.9, 16.2368) -> (-21.9, -16.2368)
  line L9 (-21.9, -16.2368) -> (-14.5891, -25.65)
  line L10 (-14.5891, -25.65) -> (-11.5, -25.65)
  line L11 (-11.5, -25.65) -> (-11.5, -20.65)
  line L12 (-11.5, -20.65) -> (11.5, -20.65)
  line L13 (11.5, -20.65) -> (11.5, -25.65)
  line L14 (11.5, -25.65) -> (14.5891, -25.65)
  line L15 (14.5891, -25.65) -> (21.9, -16.2368)
  line L16 (21.9, -16.2368) -> (21.9, 16.2368)
  line L17 (21.9, 16.2368) -> (14.5891, 25.65)
  line L18 (14.5891, 25.65) -> (11.5, 25.65)
  line L19 (11.5, 25.65) -> (11.5, 20.65)
  line L20 (11.5, 20.65) -> (-11.5, 20.65)
  line L21 (-11.5, 20.65) -> (-11.5, 25.65)
  line L22 (-11.5, 25.65) -> (-14.5891, 25.65)
  line L23 (-14.5891, 25.65) -> (-21.9, 16.2368)
  circle A0 centre (0, 15) radius 12.813
  constraint coincident L20.end A0
extrude "Extrude11" add sketch "Sketch6" along normal blind 0.2 contours L0 L1 L2 L3 L4 L5 L6 L7 L8 L9 L10 L11 L12 L13 L14 L15 L16 L17 L18 L19 L21 L22 L23 A0 bodies 3
sketch "Sketch7" plane through (0, 0, 0) normal (0, 1, 0) x (-1, 0, 0)
  line L0 (12.2821, 18.65) -> (17.4934, 18.65)
  line L1 (17.4934, 18.65) -> (19.9, 15.5514)
  line L2 (19.9, 15.5514) -> (19.9, -15.5514)
  line L3 (19.9, -15.5514) -> (17.4934, -18.65)
  line L4 (17.4934, -18.65) -> (-17.4934, -18.65)
  line L5 (-17.4934, -18.65) -> (-19.9, -15.5514)
  line L6 (-19.9, -15.5514) -> (-19.9, 15.5514)
  line L7 (-19.9, 15.5514) -> (-17.4934, 18.65)
  line L8 (-17.4934, 18.65) -> (-12.2821, 18.65)
  arc A0 (-11.5, 20.65) -> (-12.2821, 18.65) centre (0, 15) ccw
  line L9 (-11.5, 20.65) -> (-11.5, 25.65)
  line L10 (-11.5, 25.65) -> (-14.5891, 25.65)
  line L11 (-14.5891, 25.65) -> (-21.9, 16.2368)
  line L12 (-21.9, 16.2368) -> (-21.9, -16.2368)
  line L13 (-21.9, -16.2368) -> (-14.5891, -25.65)
  line L14 (-14.5891, -25.65) -> (-11.5, -25.65)
  line L15 (-11.5, -25.65) -> (-11.5, -20.65)
  line L16 (-11.5, -20.65) -> (11.5, -20.65)
  line L17 (11.5, -20.65) -> (11.5, -25.65)
  line L18 (11.5, -25.65) -> (14.5891, -25.65)
  line L19 (14.5891, -25.65) -> (21.9, -16.2368)
  line L20 (21.9, -16.2368) -> (21.9, 16.2368)
  line L21 (21.9, 16.2368) -> (14.5891, 25.65)
  line L22 (14.5891, 25.65) -> (11.5, 25.65)
  line L23 (11.5, 25.65) -> (11.5, 20.65)
  arc A1 (12.2821, 18.65) -> (11.5, 20.65) centre (0, 15) ccw
  line L24 (11.5, -20.65) -> (20, -20.65)
  line L25 (-11.5, -20.65) -> (-20, -20.65)
  line L26 (-11.5, 20.65) -> (-22, 20.65)
  line L27 (11.5, 20.65) -> (21.3505, 20.65)
  line L28 (18.6967, -17.1007) -> (18.6967, -14.6007)
  line L29 (18.6967, -14.6007) -> (20.5, -14.6007)
  line L30 (-18.6967, -17.1007) -> (-18.6967, -14.6007)
  line L31 (-18.6967, -14.6007) -> (-20.5, -14.6007)
  line L32 (18.6967, 17.1007) -> (18.6967, 14.6007)
  line L33 (18.6967, 14.6007) -> (20.5, 14.6007)
  line L34 (-18.6967, 17.1007) -> (-18.6967, 14.6007)
  line L35 (-18.6967, 14.6007) -> (-20.6384, 14.6007)
  dimension "d96" = 2.5
  dimension "d97" = 2.5
  dimension "d98" = 2.5
  dimension "d99" = 2.5
  constraint coincident L16.end L17.start
  constraint perpendicular L17 L24
  constraint coincident L15.end L16.start
  constraint perpendicular L15 L25
  constraint coincident A0.start L9.start
  constraint perpendicular L9 L26
  constraint coincident L23.end A1.end
  constraint perpendicular L23 L27
  constraint midpoint L3 L28.start
  constraint vertical L28
  constraint perpendicular L2 L29
  constraint midpoint L5 L30.start
  constraint perpendicular L29 L30
  constraint perpendicular L6 L31
  constraint midpoint L1 L32.start
  constraint parallel L2 L32
  constraint perpendicular L2 L33
  constraint midpoint L7 L34.start
  constraint perpendicular L33 L34
  constraint perpendicular L6 L35
  measures "d96" distance of L28.start L28.end
  measures "d97" distance of L30.start L30.end
  measures "d98" distance of L32.start L32.end
  measures "d99" distance of L34.start L34.end
extrude "Extrude12" add sketch "Sketch7" along normal blind 5 separate body contours L0 L1 L2 L3 L4 L5 L6 L7 L8 A0 L11 L12 L13 L16 L19 L20 L21 A1 L24 L25 L26 L27 | L1 L2 L32 L33 | L2 L3 L28 L29 | L5 L6 L30 L31 | L6 L7 L34 L35 makes body 9
sketch "Sketch8" plane through (0, 5, 0) normal (0, 1, 0) x (-1, 0, 0)
  line L0 (12.2821, 18.65) -> (17.4934, 18.65)
  line L1 (17.4934, 18.65) -> (18.6967, 17.1007)
  line L2 (19.9, 14.6007) -> (19.9, -14.6007)
  line L3 (18.6967, -17.1007) -> (17.4934, -18.65)
  line L4 (17.4934, -18.65) -> (-17.4934, -18.65)
  line L5 (-17.4934, -18.65) -> (-18.6967, -17.1007)
  line L6 (-19.9, -14.6007) -> (-19.9, 14.6007)
  line L7 (-18.6967, 17.1007) -> (-17.4934, 18.65)
  line L8 (-17.4934, 18.65) -> (-12.2821, 18.65)
  arc A0 (-11.5, 20.65) -> (-12.2821, 18.65) centre (0, 15) ccw
  line L9 (-11.5, 20.65) -> (-18.4725, 20.65)
  line L10 (-18.4725, 20.65) -> (-21.9, 16.2368)
  line L11 (-21.9, 16.2368) -> (-21.9, -16.2368)
  line L12 (-21.9, -16.2368) -> (-18.4725, -20.65)
  line L13 (-18.4725, -20.65) -> (18.4725, -20.65)
  line L14 (18.4725, -20.65) -> (21.9, -16.2368)
  line L15 (21.9, -16.2368) -> (21.9, 16.2368)
  line L16 (21.9, 16.2368) -> (18.4725, 20.65)
  line L17 (18.4725, 20.65) -> (11.5, 20.65)
  arc A1 (12.2821, 18.65) -> (11.5, 20.65) centre (0, 15) ccw
  line L18 (18.4725, 20.65) -> (-18.4725, 20.65)
  line L19 (-17.4934, 18.65) -> (17.4934, 18.65)
  line L20 (-15.95, 5.05) -> (-16.15, 5.05)
  line L21 (-16.15, 5.05) -> (-16.15, 5.25)
  line L22 (-16.15, 5.25) -> (-15.95, 5.25)
  line L23 (-15.95, 5.25) -> (-15.95, 5.05)
  line L24 (15.95, -5.15) -> (16.15, -5.15)
  line L25 (16.15, -5.15) -> (16.15, -5.35)
  line L26 (16.15, -5.35) -> (15.95, -5.35)
  line L27 (15.95, -5.35) -> (15.95, -5.15)
  line L28 (16.15, -5.35) -> (-16.15, -5.35)
  line L29 (-16.15, -5.35) -> (-16.15, 5.25)
  line L30 (-16.15, 5.25) -> (16.15, 5.25)
  line L31 (16.15, 5.25) -> (16.15, -5.35)
  line L32 (18.6967, 17.1007) -> (18.6967, 14.6007)
  line L33 (18.6967, 14.6007) -> (19.9, 14.6007)
  line L34 (19.9, -14.6007) -> (18.6967, -14.6007)
  line L35 (18.6967, -14.6007) -> (18.6967, -17.1007)
  line L36 (-18.6967, -17.1007) -> (-18.6967, -14.6007)
  line L37 (-18.6967, -14.6007) -> (-19.9, -14.6007)
  line L38 (-19.9, 14.6007) -> (-18.6967, 14.6007)
  line L39 (-18.6967, 14.6007) -> (-18.6967, 17.1007)
  dimension "d76" = 0.2
  dimension "d77" = 0.2
  dimension "d78" = 0.2
  dimension "d79" = 0.2
  constraint coincident L16.end L17.start
  constraint coincident L9.end L10.start
  constraint coincident L7.end L8.start
  constraint coincident L0.end L1.start
  constraint horizontal L20
  constraint vertical L21
  constraint horizontal L22
  constraint vertical L23
  constraint horizontal L24
  constraint vertical L25
  constraint horizontal L26
  constraint vertical L27
  constraint horizontal L28
  constraint vertical L29
  constraint horizontal L30
  constraint vertical L31
  measures "d76" distance of L20.start L20.end
  measures "d77" distance of L20.start L22.end
  measures "d78" distance of L24.start L24.end
  measures "d79" distance of L24.start L26.end
extrude "Extrude13" add sketch "Sketch8" along normal blind 2 separate body makes body 10
sketch "Sketch9" plane through (0, 10, 0) normal (0, 1, 0) x (-1, 0, 0)
  circle A0 centre (-15.75, 9.75) radius 1.665
  circle A1 centre (-15.75, 9.75) radius 1.9
  dimension "d82" = 3.8
  constraint concentric A0 A1
  measures "d82" diameter of A1
extrude "Extrude14" cut sketch "Sketch9" against normal blind 5 contours A0 | A1 bodies 10
mirror "Mirror3" about plane through (0, 0, 0) normal (1, 0, 0) of "Extrude14"
combine "Combine2" operation add target body 10 tool bodies 9
chamfer "Chamfer3" distance 1.5 angle 45 8 edges at (-21.9, 7, 0) (-20.1862, 7, -18.4434) (0, 7, -20.65) (20.1862, 7, -18.4434) (21.9, 7, 0) (20.1862, 7, 18.4434) (0, 7, 20.65) (-20.1862, 7, 18.4434) on bodies 10
extrude "Extrude15" cut 4 faces at (-15.6594, -3.7, -16.5616) (16.2333, -3.7, -16.7387) (16.1813, -3.7, 16.7824) (-16.6187, -3.7, 16.7824) along direction (0, -1, 0) blind 1 on bodies 3 bodies 3
extrude "Extrude16" cut sketch "Sketch2" against normal blind 11 contours A8 | A9 | A10 | A11 | A12 | A13 | A14 | A15 bodies 10
chamfer "Chamfer4" distance 1 angle 45 4 edges at (-17.5188, 7, -16.8839) (-17.5188, 7, 16.0161) (15.2812, 7, 16.0161) (15.2812, 7, -16.8839) on bodies 10
equation "d1 = ( 37 / 2 ) * 1 mm"
equation "d2 = ( 39.5 / 2 ) * 1 mm"
equation "d58 = ( 22 / 2 ) * 1 mm"
equation "d59 = ( 23 / 2 ) * 1 mm"
equation "d101 = ( 15.950 / 2 ) * 1 mm"
equation "d102 = ( 7.975 / 2 ) * 1 mm"
named bodies: "Board", "Case_Bottom", "Case_Top"
